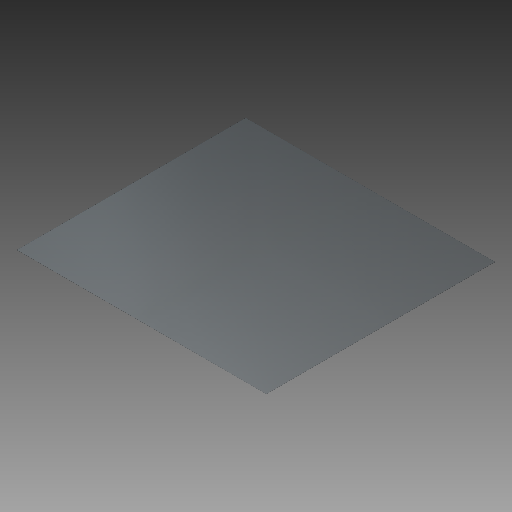
# Autodesk Inventor part: CageFloor
Saved by Autodesk Inventor 2018 (Build 220112000, 112)
## iProperties
Created: 2013-02-18
Part Number: CageFloor
Material: Generic
Document SubType Name: Modeling
Designer: Neef
Density: 1 g/cm^3
Appearance: Expanded Metal 02
Author: Neef
Autodesk Inventor part; units mm, degrees
ref_plane "YZ Plane" through (0, 0, 0) normal (1, 0, 0) x (0, 1, 0)
ref_plane "XZ Plane" through (0, 0, 0) normal (0, 1, 0) x (-1, 0, 0)
ref_plane "XY Plane" through (0, 0, 0) normal (0, 0, 1) x (1, 0, 0)
sketch "Skizze1" plane through (0, 0, 0) normal (0, 0, 1) x (1, 0, 0)
  line L0 (-300, 275) -> (300, 275)
  line L1 (300, 275) -> (300, -275)
  line L2 (300, -275) -> (-300, -275)
  line L3 (-300, -275) -> (-300, 275)
  point P0 (0, 0)
  dimension "d0" = 600
  dimension "d1" = 550
  dimension "d2" = 300
  dimension "d3" = 275
  constraints: 8 end point, 2 parallel, 1 horizontal, 1 perpendicular
  measures "d0" distance of L0.start L0.end
  measures "d1" distance of L2.end L0.start
  measures "d2" distance from line of L3 point (0, 0)
  measures "d3" distance from line of L0 point (0, 0)
extrude "Extrusion1" add sketch "Skizze1" along normal blind 0.8
equation "\"d2\" = 0.5 * d0"
equation "\"d3\" = 0.5 * d1"
